revolve tool v1 (Autodesk Fusion 360 design; units mm, degrees)
Autodesk Fusion 360 part; units mm, degrees
sketch "Sketch1" plane through (0, 0, 0) normal (0, 1, 0) x (1, 0, 0)
  line L0 (0, 0) -> (0, -50)
  line L1 (0, -50) -> (10, -50)
  line L2 (10, -50) -> (10, -40)
  line L3 (10, -40) -> (25, -15)
  line L4 (25, -15) -> (40, -10)
  line L5 (40, -10) -> (40, 0)
  line L6 (40, 0) -> (0, 0)
  dimension "d1" = 10
  dimension "d2" = 10
  dimension "d3" = 50
  dimension "d4" = 29.1548
  dimension "d5" = 15
  dimension "d6" = 139.399
  dimension "d7" = 149.036
  constraint coincident L0.start L6.end
  constraint vertical L0
  constraint perpendicular L0 L1
  constraint perpendicular L1 L2
  constraint parallel L2 L5
  constraint perpendicular L0 L6
  measures "d1" distance of L0.end L1.end
  measures "d2" distance of L4.end L5.end
  measures "d3" distance of L0.start L0.end
  measures "d4" distance of L2.end L3.end
  measures "d5" horizontal distance of L3.end L4.end
  measures "d6" angle of L3 L4
  measures "d7" angle of L2 L3
revolve "Revolve1" add sketch "Sketch1" angle 360 about axis through (0, 0, 0) along (0, 0, 1) makes body 1
sketch "Sketch2" plane through (0, 0, 0) normal (0, 1, 0) x (1, 0, 0)
  line L0 (-18, -10) -> (18, -10) construction
  line L1 (18, -10) -> (18, 10)
  line L2 (18, 10) -> (-18, 10)
  line L3 (-18, 10) -> (-18, -10)
  line L4 (-18, -10) -> (18, 10) construction
  line L5 (18, -10) -> (-18, 10) construction
  arc A0 (-18, -10) -> (18, -10) centre (0, -10) ccw
  line L6 (0, 10) -> (0, -28)
  dimension "d9" = 36
  dimension "d10" = 20
  constraint horizontal L0
  constraint perpendicular L0 L1
  constraint parallel L0 L2
  constraint parallel L1 L3
  constraint coincident L4 origin
  constraint coincident L5 origin
  constraint tangent L3 A0
  constraint midpoint L2 L6.start
  constraint midpoint A0 L6.end
  measures "d9" distance of L1.end L2.end
  measures "d10" distance of L0.end L1.end
revolve "Revolve2" add sketch "Sketch2" angle 360 about axis through (0, 0, -10) along (0, 0, 1) separate body contours L1 L2 A0 L6 makes body 2
move_body "Move1" bodies 2 to x (1, 0, 0) y (0, 1, 0) z (0, 0, 1) at (75, 0, 0)
move_body "Move2" bodies 2 to x (1, 0, 0) y (0, 1, 0) z (0, 0, 1) at (0, 0, 10)
